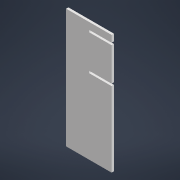
# Autodesk Inventor part: Stand
Saved by Autodesk Inventor 2021.3 (Build 253353000, 353)
## iProperties
Created: 2019-07-01
Part Number: Stand
Material: Generic
Document SubType Name: Modeling
Designer: eugen
Density: 1 g/cm^3
Appearance: Default
Author: eugen
Autodesk Inventor part; units mm, degrees
ref_plane "YZ Plane" through (0, 0, 0) normal (1, 0, 0) x (0, 1, 0)
ref_plane "XZ Plane" through (0, 0, 0) normal (0, 1, 0) x (-1, 0, 0)
ref_plane "XY Plane" through (0, 0, 0) normal (0, 0, 1) x (1, 0, 0)
sketch "Sketch1" plane through (0, 0, 0) normal (0, 0, 1) x (1, 0, 0)
  line L0 (0, 0) -> (114.3, 0)
  line L1 (114.3, 157.48) -> (114.3, 333.502)
  line L2 (114.3, 333.502) -> (0, 333.502)
  line L3 (0, 333.502) -> (0, 157.48)
  line L4 (58.42, 314.452) -> (114.3, 314.452)
  line L5 (114.3, 314.452) -> (114.3, 308.61)
  line L6 (114.3, 308.61) -> (58.42, 308.61)
  line L7 (57.15, 309.88) -> (57.15, 313.182)
  line L8 (58.42, 215.392) -> (114.3, 215.392)
  line L9 (114.3, 215.392) -> (114.3, 209.55)
  line L10 (114.3, 209.55) -> (58.42, 209.55)
  line L11 (57.15, 210.82) -> (57.15, 214.122)
  line L12 (114.3, 208.28) -> (114.3, 202.438)
  line L13 (0, 152.4) -> (114.3, 152.4) construction
  line L14 (0, 157.48) -> (0, 0)
  line L15 (114.3, 157.48) -> (114.3, 0)
  line L16 (12.7, 0) -> (18.542, 0)
  arc A0 (58.42, 314.452) -> (57.15, 313.182) centre (58.42, 313.182) ccw
  arc A1 (57.15, 309.88) -> (58.42, 308.61) centre (58.42, 309.88) ccw
  arc A2 (58.42, 215.392) -> (57.15, 214.122) centre (58.42, 214.122) ccw
  arc A3 (57.15, 210.82) -> (58.42, 209.55) centre (58.42, 210.82) ccw
  point P0 (57.15, 314.452)
  point P1 (57.15, 308.61)
  point P2 (57.15, 215.392)
  point P3 (57.15, 209.55)
  point P4 (114.3, 209.55)
  point P5 (114.3, 215.392)
  point P6 (127, 152.4)
  dimension "d1" = 5.842
  dimension "d7" = 114.3
  dimension "d8" = 5.842
  dimension "d27" = 152.4
  dimension "d30" = 99.06
  dimension "d32" = 19.05
  dimension "d33" = 57.15
  dimension "d37" = 209.55
  dimension "d38" = 1.27
  dimension "d39" = 1.27
  constraints: 34 end point, 12 point on line, 8 point on circle, 8 tangent, 6 parallel, 5 collinear, 5 horizontal, 4 centre point, 3 perpendicular, 2 equal radius, 2 vertical
  measures "d1" distance of L4.end L5.end
  measures "d7" distance between parallel lines of L1 L3
  measures "d8" distance of L8.end L9.end
  measures "d27" distance from line of L0 L13.start
  measures "d30" distance between parallel lines of L10 L6
  measures "d32" distance between parallel lines of L2 L4
  measures "d33" distance between parallel lines of L3 L11
  measures "d37" distance between parallel lines of L10 L0
  measures "d38" radius of A0
  measures "d39" radius of A1
extrude "Extrusion1" add sketch "Sketch1" along normal blind 6.35 contours L14 L3 L2 L1 L4 A0 L7 A1 L6 L8 A2 L11 A3 L10 L15 L0
equation "\"d33\" = 0.5 * d7"
body "Solid1"
